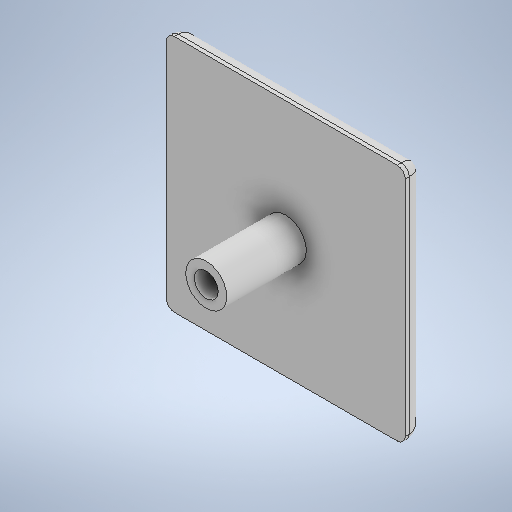
# Autodesk Inventor part: záslepka
Saved by Autodesk Inventor 2025 (Build 290162000, 162)
## iProperties
Created: 2025-01-12
Part Number: záslepka
Material: Všeobecné
Document SubType Name: Modeling
Designer: lukas
Density: 1 g/cm^3
Appearance: Výchozí
Author: lukas
Autodesk Inventor part; units mm, degrees
ref_plane "YZ Plane" through (0, 0, 0) normal (1, 0, 0) x (0, 1, 0)
ref_plane "XZ Plane" through (0, 0, 0) normal (0, 1, 0) x (-1, 0, 0)
ref_plane "XY Plane" through (0, 0, 0) normal (0, 0, 1) x (1, 0, 0)
sketch "Náčrt1" plane through (0, 0, 0) normal (0, 0, 1) x (1, 0, 0)
  line L0 (0, 21) -> (0, -21) projected
  line L1 (-21, 0) -> (21, 0) projected
  line L2 (-15, 15) -> (15, 15)
  line L3 (15, 15) -> (15, -15)
  line L4 (15, -15) -> (-15, -15)
  line L5 (-15, -15) -> (-15, 15)
  point P0 (0, 0)
  dimension "d0" = 30
  dimension "d1" = 30
  constraints: 8 end point, 2 parallel, 1 horizontal, 1 perpendicular, 2 other
  measures "d0" distance of L3.end L4.end
  measures "d1" distance of L2.end L3.end
extrude "Vysunutí1" add sketch "Náčrt1" along normal blind 2.5
sketch "Náčrt2" plane through (0, 0, 2.5) normal (0, 0, 1) x (1, 0, 0)
  line L0 (-15, -15) -> (15, -15) projected
  line L1 (15, -15) -> (15, 15) projected
  line L2 (15, 15) -> (-15, 15) projected
  line L3 (-15, 15) -> (-15, -15) projected
  line L4 (0, 21) -> (0, -21) projected
  line L5 (-21, 0) -> (21, 0) projected
  circle A0 centre (0, 0) radius 2.575
  circle A1 centre (0, 0) radius 1.5
  dimension "d5" = 5.15
  dimension "d6" = 3
  constraints: 2 centre point, 2 coincident
  measures "d5" diameter of A0
  measures "d6" diameter of A1
extrude "Vysunutí2" add sketch "Náčrt2" along normal blind 10 contours A0 L5 A1 L4 | L4 A1 L5 A0 | A0 L4 A1 L5 | L5 A1 L4 A0
fillet "Zaoblení1" radius 2 4 edges at (15, 0, 0) (0, 15, 0) (-15, 0, 0) (0, -15, 0)
fillet "Zaoblení2" radius 1 8 edges at (15, -15, 2.25) (14.4142, -14.4142, 0.5858) (15, 15, 2.25) (14.4142, 14.4142, 0.5858) (-15, 15, 2.25) (-14.4142, 14.4142, 0.5858) (-15, -15, 2.25) (-14.4142, -14.4142, 0.5858)
